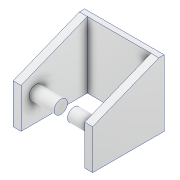
# Autodesk Inventor part: castor_link2
Saved by Autodesk Inventor 2020 (Build 240168000, 168)
## iProperties
Created: 2020-09-08
Part Number: castor_link2
Material: 알루미늄 6061
Document SubType Name: Modeling
Designer: 이호석
Mass: 13.3693 g
Surface Area: 43.0142 cm^2
Volume: 4.9516 cm^3
Density: 2.7 g/cm^3
Appearance: 알루미늄 - 평지
Author: 이호석
Autodesk Inventor part; units mm, degrees
ref_plane "YZ Plane" through (0, 0, 0) normal (1, 0, 0) x (0, 1, 0)
ref_plane "XZ Plane" through (0, 0, 0) normal (0, 1, 0) x (-1, 0, 0)
ref_plane "XY Plane" through (0, 0, 0) normal (0, 0, 1) x (1, 0, 0)
sketch "스케치1" plane through (0, 0, 0) normal (0, 0, 1) x (1, 0, 0)
  line L0 (15, -15) -> (-15, -15)
  line L1 (-15, -15) -> (-15, 15)
  line L2 (-15, 15) -> (15, 15)
  line L3 (15, 15) -> (15, -15)
  line L4 (15, -15) -> (-15, 15) construction
  line L5 (-15, -15) -> (15, 15) construction
  point P0 (0, 0)
  dimension "d0" = 30
  dimension "d1" = 30
  constraints: 12 end point, 2 midpoint, 2 parallel, 1 horizontal, 1 perpendicular
  measures "d0" distance of L1.end L2.end
  measures "d1" distance of L0.end L1.end
extrude "돌출1" add sketch "스케치1" along normal blind 2
sketch "스케치2" plane through (0, 0, 2) normal (0, 0, 1) x (1, 0, 0)
  line L0 (-15, 15) -> (-15, -15) projected
  line L1 (-15, -15) -> (15, -15) projected
  line L2 (-15, 15) -> (-12, 15)
  line L3 (-12, 15) -> (-12, -15)
  line L4 (-12, -15) -> (-15, -15)
  line L5 (-15, -15) -> (-15, 15)
  line L6 (15, -15) -> (15, 15) projected
  line L7 (15, 15) -> (12, 15)
  line L8 (12, 15) -> (12, -15)
  line L9 (12, -15) -> (15, -15)
  line L10 (15, -15) -> (15, 15)
  point P0 (0, 0)
  dimension "d4" = 3
  dimension "d5" = 3
  constraints: 16 end point, 4 parallel, 2 horizontal, 2 perpendicular, 2 point on line
  measures "d4" distance of L3.end L4.end
  measures "d5" distance of L9.end L8.end
extrude "돌출2" add sketch "스케치2" along normal blind 30
sketch "스케치3" plane through (0, 0, 0) normal (0, 0, -1) x (-1, 0, 0)
  circle A0 centre (0, 0) radius 5
  dimension "d8" = 10
  constraints: 1 centre point, 1 coincident
  measures "d8" diameter of A0
extrude "돌출3" add sketch "스케치3" along normal blind 1
sketch "스케치4" plane through (15, -15, 0) normal (1, 0, 0) x (0, 0, -1)
  line L0 (0, 0) -> (-39, 0)
  line L1 (-39, 0) -> (-26.5, 0)
  line L2 (-2, 0) -> (-32, 0) projected
  line L3 (-26.5, 0) -> (-26.5, 10)
  circle A0 centre (-26.5, 10) radius 2.5
  line L4 (0, 0) -> (-32, 0) projected
  line L5 (0, 0) -> (-34, 0)
  line L6 (-34, 0) -> (-21.5, 0)
  line L7 (-21.5, 0) -> (-21.5, 10)
  circle A1 centre (-21.5, 10) radius 2.5
  point P0 (0, 15)
  dimension "d11" = 39
  dimension "d12" = 12.5
  dimension "d13" = 5
  dimension "d14" = 10
  dimension "d32" = 34
  dimension "d33" = 12.5
  constraints: 12 end point, 3 point on line, 2 centre point, 2 coincident, 2 perpendicular, 1 equal radius, 1 horizontal
  measures "d11" distance of L0.start L0.end
  measures "d12" distance of L0.end L1.end
  measures "d13" diameter of A0
  measures "d14" distance of L1.end L3.end
  measures "d32" distance of L0.start L5.end
  measures "d33" distance of L5.end L6.end
extrude "돌출4" add sketch "스케치4" against normal blind 12.5 contours A1
sketch "스케치5" plane through (-15, -15, 0) normal (-1, 0, 0) x (0, 0, 1)
  circle A0 centre (26.5, 10) radius 2.5 projected
  circle A1 centre (21.5, 10) radius 2.5 projected
  circle A2 centre (21.5, 10) radius 2.5 projected
  point P0 (0, 15)
extrude "돌출5" add sketch "스케치5" against normal blind 12.5 contours A1
sketch "스케치6" plane through (15, -15, 0) normal (1, 0, 0) x (0, 0, -1)
  line L0 (0, 30) -> (-32, 30) projected
  line L1 (-2, 30) -> (-32, 30) projected
  line L2 (-2, 30) -> (-32, 30) projected
  line L3 (0, 30) -> (-32, 30) projected
  line L4 (-2, 0) -> (-2, 30) projected
  line L5 (-2, 30) -> (-2, 0) projected
  line L6 (0, 30) -> (-32, 30) projected
  line L7 (-2, 30) -> (-2, 0) projected
  line L8 (0, 30) -> (-2, 30)
  line L9 (-2, 30) -> (-7, 30)
  line L10 (-2, 30) -> (-32, 30) projected
  line L11 (-32, 0) -> (-32, 30) projected
  line L12 (-7, 30) -> (-32, 30)
  line L13 (-32, 30) -> (-32, 20)
  line L14 (-32, 20) -> (-7, 30)
  circle A0 centre (-26.5, 10) radius 2.5 projected
  line L15 (0, 0) -> (-32, 0) projected
  line L16 (-32, 0) -> (-27, 0)
  line L17 (-27, 0) -> (-27, 22)
  point P0 (0, 15)
  point P1 (-7, 30)
  dimension "d19" = 2
  dimension "d20" = 5
  dimension "d21" = 10
  dimension "d22" = 5
  constraints: 14 end point, 3 point on line, 1 collinear, 1 horizontal, 1 perpendicular, 3 other
  measures "d19" distance of L3.start L1.start
  measures "d20" distance of L5.start L9.end
  measures "d21" distance of L0.end L13.end
  measures "d22" distance of L11.start L16.end
extrude "돌출6" cut sketch "스케치6" against normal through all contours L14 L11 L0 | L17 A0 L15 L11 L14 | L17 A0 picked at (-27.6602, 9.8965)
sketch "스케치7" plane through (15, -15, 0) normal (1, 0, 0) x (0, 0, -1)
  line L0 (-2, 0) -> (-2, 30) projected
  line L1 (-2, 30) -> (-2, 25)
  line L2 (-2, 30) -> (-2, 0) projected
  line L3 (-2, 25) -> (-27, 25)
  line L4 (-27, 22) -> (-27, 0) projected
  arc A0 (-27, 7.5505) -> (-27, 12.4495) centre (-26.5, 10) ccw projected
  line L5 (-27, 25) -> (-27, 15)
  line L6 (-27, 15) -> (-2, 25)
  line L7 (-27, 22) -> (-27, 0) projected
  line L8 (0, 0) -> (-27, 0) projected
  line L9 (0, 0) -> (0, 30) projected
  line L10 (0, 30) -> (-7, 30) projected
  line L11 (-7, 30) -> (-27, 22) projected
  point P0 (0, 15)
  point P1 (-2, 25)
  dimension "d25" = 5
  dimension "d26" = 10
  constraints: 8 end point, 2 point on line, 1 perpendicular
  measures "d25" distance of L0.end L1.end
  measures "d26" distance of L3.end L5.end
extrude "돌출7" cut sketch "스케치7" against normal through all contours L3 L11 L10 L0 | L6 L4 L11 L3
sketch "스케치8" plane through (15, -15, 0) normal (1, 0, 0) x (0, 0, -1)
  line L0 (0, 0) -> (0, 30) projected
  line L1 (0, 30) -> (0, 25)
  line L2 (0, 25) -> (-2, 25)
  line L3 (0, 30) -> (-2, 30) projected
  line L4 (-2, 25) -> (-2, 30)
  line L5 (0, 30) -> (-2, 30)
  point P0 (0, 15)
  dimension "d29" = 5
  constraints: 8 end point, 1 collinear, 1 point on line
  measures "d29" distance of L0.end L1.end
extrude "돌출8" cut sketch "스케치8" against normal through all
